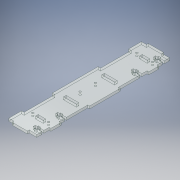
# Autodesk Inventor part: Cubierta_Rodamientos
Saved by Autodesk Inventor 2019 (Build 230136000, 136)
## iProperties
Created: 2020-04-04
Part Number: Cubierta_Rodamientos
Material: Generic
Document SubType Name: Modeling
Designer: Jurgen
Density: 1 g/cm^3
Appearance: Clear
Mass: 67.373 g
Surface Area: 309.762 cm^2
Volume: 67.373 cm^3
Author: Jurgen
Autodesk Inventor part; units mm, degrees
ref_plane "YZ Plane" through (0, 0, 0) normal (1, 0, 0) x (0, 1, 0)
ref_plane "XZ Plane" through (0, 0, 0) normal (0, 1, 0) x (-1, 0, 0)
ref_plane "XY Plane" through (0, 0, 0) normal (0, 0, 1) x (1, 0, 0)
sketch "Sketch1" plane through (0, 0, 0) normal (0, 1, 0) x (-1, 0, 0)
  line L0 (-25, -130) -> (25, -130)
  line L1 (25, 130) -> (-25, 130)
  line L2 (-25, 130) -> (-25, -130)
  line L3 (-25, -130) -> (25, 130) construction
  line L4 (25, -130) -> (-25, 130) construction
  line L5 (25, 130) -> (30, 130)
  line L6 (30, 130) -> (30, 105)
  line L7 (30, 105) -> (25, 105)
  line L8 (25, -130) -> (30, -130)
  line L9 (30, -130) -> (30, -105)
  line L10 (30, -105) -> (25, -105)
  line L11 (25, 105) -> (-25, 105) construction
  line L12 (3.2055, 0) -> (-25, 0) construction
  line L13 (25, -105) -> (-25, -105) construction
  line L14 (25, 45) -> (30, 45)
  line L15 (30, 45) -> (30, -45)
  line L16 (30, -45) -> (25, -45)
  line L17 (25, -105) -> (25, -45)
  line L18 (25, 45) -> (25, 105)
  point P0 (0, 0)
  dimension "d0" = 50
  dimension "d1" = 260
  dimension "d2" = 5
  dimension "d3" = 25
  dimension "d4" = 5
  dimension "d5" = 25
  dimension "d7" = 5
  dimension "d8" = 90
  dimension "d29" = 60
  dimension "d30" = 60
  constraints: 38 end point, 9 perpendicular, 5 parallel, 3 horizontal, 3 midpoint, 2 point on line
  measures "d0" distance of L1.end L1.start
  measures "d1" distance of L1.start L0.end
  measures "d2" distance of L7.end L6.end
  measures "d3" distance of L5.end L6.end
  measures "d4" distance of L10.end L9.end
  measures "d5" distance of L9.end L8.end
  measures "d7" distance of L14.start L14.end
  measures "d8" distance of L14.end L15.end
  measures "d29" distance of L10.end L16.end
  measures "d30" distance of L14.start L7.end
extrude "Extrusion1" add sketch "Sketch1" along normal blind 5
sketch "Sketch2" plane through (0, 5, 0) normal (0, 1, 0) x (1, 0, 0)
  line L0 (25, 130) -> (-30, 130) construction
  line L1 (-30, 130) -> (-30, 105) construction
  line L2 (-30, 105) -> (-25, 105) construction
  line L3 (-25, 105) -> (-25, 45) construction
  line L4 (-25, 45) -> (-30, 45) construction
  line L5 (-30, 45) -> (-30, -45) construction
  line L6 (-30, -45) -> (-25, -45) construction
  line L7 (-25, -45) -> (-25, -105) construction
  line L8 (-25, -105) -> (-30, -105) construction
  line L9 (-30, -105) -> (-30, -130) construction
  line L10 (-30, -130) -> (25, -130) construction
  line L11 (25, -130) -> (25, 130) construction
  line L12 (-30, 45) -> (-30, -45) construction
  line L13 (25, -130) -> (25, 130) construction
  line L14 (7.5, -100) -> (-7.5, -100)
  line L15 (-7.5, -100) -> (-7.5, -95)
  line L16 (-7.5, -95) -> (7.5, -95)
  line L17 (7.5, -95) -> (7.5, -100)
  line L18 (7.5, 109) -> (-7.5, 109)
  line L19 (-7.5, 109) -> (-7.5, 104)
  line L20 (-7.5, 104) -> (7.5, 104)
  line L21 (7.5, 104) -> (7.5, 109)
  line L22 (-7.5, 106.5) -> (25, 106.5) construction
  line L23 (-7.5, 106.5) -> (-30, 106.5) construction
  circle A0 centre (-15.5, 106.5) radius 2
  circle A1 centre (15.5, 106.5) radius 2
  line L24 (-7.5, -97.5) -> (25, -97.5) construction
  line L25 (-7.5, -97.5) -> (-25, -97.5) construction
  circle A2 centre (-15.5, -97.5) radius 2
  circle A3 centre (15.5, -97.5) radius 2
  point P0 (0, 0)
  dimension "d11" = 15
  dimension "d12" = 5
  dimension "d13" = 35
  dimension "d14" = 17.5
  dimension "d17" = 5
  dimension "d18" = 15
  dimension "d19" = 26
  dimension "d31" = 17.5
  dimension "d32" = 4
  dimension "d33" = 4
  dimension "d34" = 8
  dimension "d35" = 8
  dimension "d36" = 4
  dimension "d37" = 4
  dimension "d38" = 8
  dimension "d39" = 8
  constraints: 24 end point, 10 point on line, 4 centre point, 3 perpendicular, 2 midpoint, 2 parallel, 1 horizontal
  measures "d11" distance of L15.end L16.end
  measures "d12" distance of L14.end L15.end
  measures "d13" distance between parallel lines of L10 L16
  measures "d14" distance between parallel lines of L11 L17
  measures "d17" distance of L20.end L21.end
  measures "d18" distance of L20.start L20.end
  measures "d19" distance between parallel lines of L0 L20
  measures "d31" distance between parallel lines of L11 L21
  measures "d32" diameter of A0
  measures "d33" diameter of A1
  measures "d34" distance from line of L19 A0.centre
  measures "d35" distance from line of A1.centre L21
  measures "d36" diameter of A2
  measures "d37" diameter of A3
  measures "d38" distance from line of L15 A2.centre
  measures "d39" distance from line of A3.centre L17
extrude "Extrusion2" cut sketch "Sketch2" against normal blind 5
sketch "Sketch3" plane through (0, 5, 0) normal (0, 1, 0) x (1, 0, 0)
  line L0 (7.5, -95) -> (7.5, -100) construction
  line L1 (7.5, -100) -> (-7.5, -100) construction
  line L2 (-7.5, -100) -> (-7.5, -95) construction
  line L3 (-7.5, -95) -> (7.5, -95) construction
  line L4 (7.5, 104) -> (-7.5, 104) construction
  line L5 (-7.5, 104) -> (-7.5, 109) construction
  line L6 (-7.5, 109) -> (7.5, 109) construction
  line L7 (7.5, 109) -> (7.5, 104) construction
  line L8 (25, 130) -> (-30, 130) construction
  line L9 (-30, 130) -> (-30, 105) construction
  line L10 (-30, 105) -> (-25, 105) construction
  line L11 (-25, 105) -> (-25, 45) construction
  line L12 (-25, 45) -> (-30, 45) construction
  line L13 (-30, 45) -> (-30, -45) construction
  line L14 (-30, -45) -> (-25, -45) construction
  line L15 (-25, -45) -> (-25, -105) construction
  line L16 (-25, -105) -> (-30, -105) construction
  line L17 (-30, -105) -> (-30, -130) construction
  line L18 (-30, -130) -> (25, -130) construction
  line L19 (25, -130) -> (25, 130) construction
  circle A0 centre (-5, 15) radius 2
  circle A1 centre (-5, -15) radius 2
  line L20 (-30, 45) -> (-30, -45) construction
  line L21 (-30, 0) -> (25, 0) construction
  point P0 (0, 0)
  dimension "d20" = 4
  dimension "d21" = 4
  dimension "d23" = 15
  dimension "d24" = 15
  dimension "d25" = 25
  dimension "d26" = 25
  constraints: 2 centre point, 2 end point, 2 midpoint
  measures "d20" diameter of A0
  measures "d21" diameter of A1
  measures "d23" distance from line of A0.centre L21
  measures "d24" vertical distance of L21.start A1.centre
  measures "d25" distance from line of L13 A0.centre
  measures "d26" distance from line of A1.centre L13
extrude "Extrusion3" cut sketch "Sketch3" against normal blind 5
sketch "Sketch4" plane through (0, 5, 0) normal (0, 1, 0) x (1, 0, 0)
  circle A0 centre (-5, 15) radius 2 construction
  circle A1 centre (-5, -15) radius 2 construction
  line L0 (7.5, -95) -> (7.5, -100) construction
  line L1 (7.5, -100) -> (-7.5, -100) construction
  line L2 (-7.5, -100) -> (-7.5, -95) construction
  line L3 (-7.5, -95) -> (7.5, -95) construction
  circle A2 centre (-15.5, -97.5) radius 2 construction
  circle A3 centre (-15.5, 106.5) radius 2 construction
  circle A4 centre (15.5, 106.5) radius 2 construction
  circle A5 centre (15.5, -97.5) radius 2 construction
  line L4 (7.5, 104) -> (-7.5, 104) construction
  line L5 (-7.5, 104) -> (-7.5, 109) construction
  line L6 (-7.5, 109) -> (7.5, 109) construction
  line L7 (7.5, 109) -> (7.5, 104) construction
  line L8 (25, 130) -> (-30, 130) construction
  line L9 (-30, 130) -> (-30, 105) construction
  line L10 (-30, 105) -> (-25, 105) construction
  line L11 (-25, 105) -> (-25, 45) construction
  line L12 (-25, 45) -> (-30, 45) construction
  line L13 (-30, 45) -> (-30, -45) construction
  line L14 (-30, -45) -> (-25, -45) construction
  line L15 (-25, -45) -> (-25, -105) construction
  line L16 (-25, -105) -> (-30, -105) construction
  line L17 (-30, -105) -> (-30, -130) construction
  line L18 (-30, -130) -> (25, -130) construction
  line L19 (25, -130) -> (25, 130) construction
  line L20 (0, 0) -> (0, -130) construction
  line L21 (-30, -130) -> (25, -130) construction
  line L22 (0, 0) -> (0, 130) construction
  line L23 (25, 130) -> (-30, 130) construction
  line L24 (25, 0) -> (-30, 0) construction
  line L25 (-30, 45) -> (-30, -45) construction
  line L26 (12.5, 40) -> (-12.5, 40)
  line L27 (-12.5, 40) -> (-12.5, 35)
  line L28 (-12.5, 35) -> (12.5, 35)
  line L29 (12.5, 35) -> (12.5, 40)
  line L30 (12.5, 40) -> (-12.5, 35) construction
  line L31 (-12.5, 40) -> (12.5, 35) construction
  line L32 (12.5, -40) -> (-12.5, -40)
  line L33 (-12.5, -40) -> (-12.5, -35)
  line L34 (-12.5, -35) -> (12.5, -35)
  line L35 (12.5, -35) -> (12.5, -40)
  line L36 (12.5, -40) -> (-12.5, -35) construction
  line L37 (-12.5, -40) -> (12.5, -35) construction
  point P0 (0, 37.5)
  point P1 (0, -37.5)
  dimension "d42" = 25
  dimension "d43" = 5
  dimension "d44" = 90
  constraints: 30 end point, 6 midpoint, 5 symmetric about line, 4 point on line, 2 parallel, 2 perpendicular, 1 horizontal
  measures "d42" distance of L28.end L27.end
  measures "d43" distance of L27.end L26.end
  measures "d44" distance between parallel lines of L8 L26
extrude "Extrusion4" cut sketch "Sketch4" against normal blind 10
sketch "Sketch5" plane through (0, 5, 0) normal (0, 1, 0) x (1, 0, 0)
  line L0 (-12.5, 35) -> (-12.5, 40) construction
  line L1 (-12.5, 40) -> (12.5, 40) construction
  line L2 (12.5, 40) -> (12.5, 35) construction
  line L3 (12.5, 35) -> (-12.5, 35) construction
  line L4 (12.5, -40) -> (-12.5, -40) construction
  line L5 (-12.5, -40) -> (-12.5, -35) construction
  line L6 (-12.5, -35) -> (12.5, -35) construction
  line L7 (12.5, -35) -> (12.5, -40) construction
  circle A0 centre (-5, 15) radius 2 construction
  circle A1 centre (-5, -15) radius 2 construction
  line L8 (7.5, -95) -> (7.5, -100) construction
  line L9 (7.5, -100) -> (-7.5, -100) construction
  line L10 (-7.5, -100) -> (-7.5, -95) construction
  line L11 (-7.5, -95) -> (7.5, -95) construction
  circle A2 centre (-15.5, -97.5) radius 2 construction
  circle A3 centre (-15.5, 106.5) radius 2 construction
  circle A4 centre (15.5, 106.5) radius 2 construction
  circle A5 centre (15.5, -97.5) radius 2 construction
  line L12 (7.5, 104) -> (-7.5, 104) construction
  line L13 (-7.5, 104) -> (-7.5, 109) construction
  line L14 (-7.5, 109) -> (7.5, 109) construction
  line L15 (7.5, 109) -> (7.5, 104) construction
  line L16 (25, 130) -> (-30, 130) construction
  line L17 (-30, 130) -> (-30, 105) construction
  line L18 (-30, 105) -> (-25, 105) construction
  line L19 (-25, 105) -> (-25, 45) construction
  line L20 (-25, 45) -> (-30, 45) construction
  line L21 (-30, 45) -> (-30, -45) construction
  line L22 (-30, -45) -> (-25, -45) construction
  line L23 (-25, -45) -> (-25, -105) construction
  line L24 (-25, -105) -> (-30, -105) construction
  line L25 (-30, -105) -> (-30, -130) construction
  line L26 (-30, -130) -> (25, -130) construction
  line L27 (25, -130) -> (25, 130) construction
  line L28 (0, -40) -> (0, -45) construction
  line L29 (0, -45) -> (-20, -45) construction
  line L30 (-20, -45) -> (-20, -40) construction
  line L31 (-20, -40) -> (0, -40) construction
  line L32 (0, 45) -> (0, 40) construction
  line L33 (0, 40) -> (-20, 40) construction
  line L34 (-20, 40) -> (-20, 45) construction
  line L35 (-20, 45) -> (0, 45) construction
  circle A6 centre (-30.5, 97.5) radius 2 construction
  circle A7 centre (-30.5, -106.5) radius 2 construction
  circle A8 centre (10.5, -106.5) radius 2 construction
  circle A9 centre (10.5, 97.5) radius 2 construction
  line L36 (-22.5, 95) -> (-22.5, 100) construction
  line L37 (-22.5, 100) -> (2.5, 100) construction
  line L38 (2.5, 100) -> (2.5, 95) construction
  line L39 (2.5, 95) -> (-22.5, 95) construction
  line L40 (2.5, -109) -> (-22.5, -109) construction
  line L41 (-22.5, -109) -> (-22.5, -104) construction
  line L42 (-22.5, -104) -> (2.5, -104) construction
  line L43 (2.5, -104) -> (2.5, -109) construction
  line L44 (-50, -130) -> (25, -130) construction
  line L45 (25, -130) -> (25, 130) construction
  line L46 (25, 130) -> (-50, 130) construction
  line L47 (-50, 130) -> (-50, 105) construction
  line L48 (-50, 105) -> (-45, 105) construction
  line L49 (-45, 105) -> (-45, 45) construction
  line L50 (-45, 45) -> (-50, 45) construction
  line L51 (-50, 45) -> (-50, -45) construction
  line L52 (-50, -45) -> (-45, -45) construction
  line L53 (-45, -45) -> (-45, -105) construction
  line L54 (-45, -105) -> (-50, -105) construction
  line L55 (-50, -105) -> (-50, -130) construction
  line L56 (25, -130) -> (25, 130) construction
  line L57 (25, -120) -> (10, -120) construction
  line L58 (10, -120) -> (10, -116) construction
  line L59 (10, -116) -> (25, -116) construction
  line L60 (25, -116) -> (25, -120) construction
  line L61 (10, -118) -> (25, -118) construction
  line L62 (18, -114) -> (14, -114) construction
  line L63 (14, -114) -> (14, -122) construction
  line L64 (14, -122) -> (18, -122) construction
  line L65 (18, -122) -> (18, -114) construction
  line L66 (18, -114) -> (14, -122) construction
  line L67 (14, -114) -> (18, -122) construction
  line L68 (25, -116) -> (25, -120)
  line L69 (25, -120) -> (18, -120)
  line L70 (18, -120) -> (18, -122)
  line L71 (18, -122) -> (14, -122)
  line L72 (14, -122) -> (14, -120)
  line L73 (14, -120) -> (10, -120)
  line L74 (10, -120) -> (10, -116)
  line L75 (10, -116) -> (14, -116)
  line L76 (14, -116) -> (14, -114)
  line L77 (14, -114) -> (18, -114)
  line L78 (18, -114) -> (18, -116)
  line L79 (18, -116) -> (25, -116)
  line L80 (18, -70) -> (14, -70) construction
  line L81 (14, -70) -> (18, -70)
  line L82 (18, -70) -> (18, -72)
  line L83 (10, -72) -> (25, -72) construction
  line L84 (10, -74) -> (25, -74) construction
  line L85 (25, -76) -> (10, -76) construction
  line L86 (18, -78) -> (18, -70) construction
  line L87 (18, -70) -> (14, -78) construction
  line L88 (14, -70) -> (18, -78) construction
  line L89 (14, -70) -> (14, -78) construction
  line L90 (14, -78) -> (18, -78) construction
  line L91 (18, -78) -> (14, -78)
  line L92 (18, -76) -> (18, -78)
  line L93 (25, -76) -> (18, -76)
  line L94 (25, -72) -> (25, -76) construction
  line L95 (25, -72) -> (25, -76)
  line L96 (18, -72) -> (25, -72)
  line L97 (10, -76) -> (10, -72) construction
  line L98 (14, -78) -> (14, -76)
  line L99 (14, -72) -> (14, -70)
  line L100 (10, -72) -> (14, -72)
  line L101 (14, -76) -> (10, -76)
  line L102 (10, -76) -> (10, -72)
  line L103 (25, -106) -> (28.5, -106)
  line L104 (28.5, -106) -> (28.5, -86)
  line L105 (28.5, -86) -> (25, -86)
  line L106 (25, -86) -> (25, -106)
  line L107 (25, 106) -> (25, 86)
  line L108 (28.5, 106) -> (25, 106)
  line L109 (28.5, 86) -> (28.5, 106)
  line L110 (25, 86) -> (28.5, 86)
  line L111 (10, 72) -> (10, 76) construction
  line L112 (10, 72) -> (10, 76)
  line L113 (14, 76) -> (14, 78)
  line L114 (10, 76) -> (14, 76)
  line L115 (14, 72) -> (10, 72)
  line L116 (14, 70) -> (14, 72)
  line L117 (14, 78) -> (14, 70) construction
  line L118 (18, 72) -> (18, 70)
  line L119 (18, 70) -> (18, 78) construction
  line L120 (18, 70) -> (14, 70)
  line L121 (18, 78) -> (14, 70) construction
  line L122 (14, 78) -> (18, 70) construction
  line L123 (14, 70) -> (18, 70) construction
  line L124 (18, 78) -> (18, 76)
  line L125 (18, 78) -> (14, 78) construction
  line L126 (10, 76) -> (25, 76) construction
  line L127 (10, 74) -> (25, 74) construction
  line L128 (25, 72) -> (10, 72) construction
  line L129 (14, 78) -> (18, 78)
  line L130 (18, 122) -> (14, 122) construction
  line L131 (14, 122) -> (18, 122)
  line L132 (18, 122) -> (18, 120)
  line L133 (10, 118) -> (25, 118) construction
  line L134 (25, 116) -> (10, 116) construction
  line L135 (10, 120) -> (25, 120) construction
  line L136 (14, 114) -> (18, 114) construction
  line L137 (18, 114) -> (14, 114)
  line L138 (14, 114) -> (14, 116)
  line L139 (14, 116) -> (10, 116)
  line L140 (10, 120) -> (14, 120)
  line L141 (10, 116) -> (10, 120)
  line L142 (10, 116) -> (10, 120) construction
  line L143 (18, 114) -> (18, 122) construction
  line L144 (18, 122) -> (14, 114) construction
  line L145 (14, 122) -> (14, 114) construction
  line L146 (14, 120) -> (14, 122)
  line L147 (14, 122) -> (18, 114) construction
  line L148 (18, 76) -> (25, 76)
  line L149 (25, 76) -> (25, 72) construction
  line L150 (25, 76) -> (25, 72)
  line L151 (25, 72) -> (18, 72)
  line L152 (25, 120) -> (25, 116) construction
  line L153 (25, 120) -> (25, 116)
  line L154 (18, 120) -> (25, 120)
  line L155 (25, 116) -> (18, 116)
  line L156 (18, 116) -> (18, 114)
  line L157 (25, -30) -> (28.5, -30)
  line L158 (28.5, -30) -> (28.5, 30)
  line L159 (28.5, 30) -> (25, 30)
  line L160 (25, 30) -> (25, -30)
  line L161 (25, -130) -> (25, 130)
  point P0 (0, 0)
  point P1 (0, 0)
  point P2 (16, -118)
  point P3 (16, -74)
  point P4 (16, 74)
  point P5 (16, 118)
  dimension "d47" = 15
  dimension "d48" = 4
  dimension "d49" = 4
  dimension "d50" = 8
  dimension "d51" = 4
  dimension "d52" = 10
  dimension "d53" = 15
  dimension "d54" = 4
  dimension "d55" = 4
  dimension "d56" = 8
  dimension "d57" = 4
  dimension "d58" = 40
  dimension "d59" = 3.5
  dimension "d60" = 20
  dimension "d61" = 10
  dimension "d62" = 15
  dimension "d63" = 4
  dimension "d64" = 4
  dimension "d65" = 8
  dimension "d66" = 4
  dimension "d67" = 15
  dimension "d68" = 4
  dimension "d69" = 4
  dimension "d70" = 8
  dimension "d71" = 4
  dimension "d72" = 40
  dimension "d73" = 3.5
  dimension "d74" = 20
  dimension "d75" = 10
  dimension "d76" = 10
  dimension "d77" = 3.5
  dimension "d78" = 60
  dimension "d79" = 30
  constraints: 266 end point, 39 point on line, 23 perpendicular, 22 parallel, 16 midpoint, 11 horizontal, 9 collinear, 4 centre point, 1 vertical, 3 other
  measures "d47" distance of L58.end L59.end
  measures "d48" distance of L57.end L58.end
  measures "d49" distance of L64.end L63.end
  measures "d50" distance of L63.end L62.end
  measures "d51" distance between parallel lines of L58 L63
  measures "d52" distance between parallel lines of L44 L57
  measures "d53" distance of L83.start L83.end
  measures "d54" distance of L85.end L83.start
  measures "d55" distance of L86.start L87.end
  measures "d56" distance of L87.end L80.end
  measures "d57" distance between parallel lines of L97 L89
  measures "d58" distance between parallel lines of L79 L93
  measures "d59" distance of L105.end L104.end
  measures "d60" distance of L104.end L103.end
  measures "d61" distance between parallel lines of L59 L103
  measures "d62" distance of L111.end L126.end
  measures "d63" distance of L111.start L111.end
  measures "d64" distance of L118.end L116.start
  measures "d65" distance of L116.start L113.end
  measures "d66" distance between parallel lines of L111 L117
  measures "d67" distance of L135.start L135.end
  measures "d68" distance of L134.end L135.start
  measures "d69" distance of L136.end L136.start
  measures "d70" distance of L136.start L130.end
  measures "d71" distance between parallel lines of L142 L145
  measures "d72" distance between parallel lines of L148 L155
  measures "d73" distance of L107.start L108.start
  measures "d74" distance of L108.start L109.start
  measures "d75" distance between parallel lines of L126 L110
  measures "d76" distance between parallel lines of L46 L154
  measures "d77" distance of L159.end L158.end
  measures "d78" distance of L158.end L157.end
  measures "d79" distance from line of point (0, 0) L157
extrude "Extrusion5" add sketch "Sketch5" against normal blind 5 contours L107 L108 L109 L110 | L160 L159 L158 L157 | L106 L105 L104 L103
sketch "Sketch6" plane through (0, 5, 0) normal (0, 1, 0) x (1, 0, 0)
  line L0 (-12.5, 35) -> (-12.5, 40) construction
  line L1 (-12.5, 40) -> (12.5, 40) construction
  line L2 (12.5, 40) -> (12.5, 35) construction
  line L3 (12.5, 35) -> (-12.5, 35) construction
  line L4 (12.5, -40) -> (-12.5, -40) construction
  line L5 (-12.5, -40) -> (-12.5, -35) construction
  line L6 (-12.5, -35) -> (12.5, -35) construction
  line L7 (12.5, -35) -> (12.5, -40) construction
  circle A0 centre (-5, 15) radius 2 construction
  circle A1 centre (-5, -15) radius 2 construction
  line L8 (7.5, -95) -> (7.5, -100) construction
  line L9 (7.5, -100) -> (-7.5, -100) construction
  line L10 (-7.5, -100) -> (-7.5, -95) construction
  line L11 (-7.5, -95) -> (7.5, -95) construction
  circle A2 centre (-15.5, -97.5) radius 2 construction
  circle A3 centre (-15.5, 106.5) radius 2 construction
  circle A4 centre (15.5, 106.5) radius 2 construction
  circle A5 centre (15.5, -97.5) radius 2 construction
  line L12 (7.5, 104) -> (-7.5, 104) construction
  line L13 (-7.5, 104) -> (-7.5, 109) construction
  line L14 (-7.5, 109) -> (7.5, 109) construction
  line L15 (7.5, 109) -> (7.5, 104) construction
  line L16 (25, 130) -> (-30, 130) construction
  line L17 (-30, 130) -> (-30, 105) construction
  line L18 (-30, 105) -> (-25, 105) construction
  line L19 (-25, 105) -> (-25, 45) construction
  line L20 (-25, 45) -> (-30, 45) construction
  line L21 (-30, 45) -> (-30, -45) construction
  line L22 (-30, -45) -> (-25, -45) construction
  line L23 (-25, -45) -> (-25, -105) construction
  line L24 (-25, -105) -> (-30, -105) construction
  line L25 (-30, -105) -> (-30, -130) construction
  line L26 (-30, -130) -> (25, -130) construction
  line L27 (25, -130) -> (25, -106) construction
  line L28 (25, -106) -> (28.5, -106) construction
  line L29 (28.5, -106) -> (28.5, -86) construction
  line L30 (28.5, -86) -> (25, -86) construction
  line L31 (25, -86) -> (25, -30) construction
  line L32 (25, -30) -> (28.5, -30) construction
  line L33 (28.5, -30) -> (28.5, 30) construction
  line L34 (28.5, 30) -> (25, 30) construction
  line L35 (25, 30) -> (25, 86) construction
  line L36 (28.5, 86) -> (25, 86) construction
  line L37 (28.5, 106) -> (28.5, 86) construction
  line L38 (25, 106) -> (28.5, 106) construction
  line L39 (25, 106) -> (25, 130) construction
  line L40 (0, -40) -> (0, -45) construction
  line L41 (0, -45) -> (-20, -45) construction
  line L42 (-20, -45) -> (-20, -40) construction
  line L43 (-20, -40) -> (0, -40) construction
  line L44 (0, 45) -> (0, 40) construction
  line L45 (0, 40) -> (-20, 40) construction
  line L46 (-20, 40) -> (-20, 45) construction
  line L47 (-20, 45) -> (0, 45) construction
  circle A6 centre (-30.5, 97.5) radius 2 construction
  circle A7 centre (-30.5, -106.5) radius 2 construction
  circle A8 centre (10.5, -106.5) radius 2 construction
  circle A9 centre (10.5, 97.5) radius 2 construction
  line L48 (-22.5, 95) -> (-22.5, 100) construction
  line L49 (-22.5, 100) -> (2.5, 100) construction
  line L50 (2.5, 100) -> (2.5, 95) construction
  line L51 (2.5, 95) -> (-22.5, 95) construction
  line L52 (2.5, -109) -> (-22.5, -109) construction
  line L53 (-22.5, -109) -> (-22.5, -104) construction
  line L54 (-22.5, -104) -> (2.5, -104) construction
  line L55 (2.5, -104) -> (2.5, -109) construction
  line L56 (-50, -130) -> (25, -130) construction
  line L57 (25, -130) -> (25, -106) construction
  line L58 (25, -106) -> (30.5, -106) construction
  line L59 (30.5, -106) -> (30.5, -86) construction
  line L60 (30.5, -86) -> (23, -86) construction
  line L61 (23, -86) -> (23, -30) construction
  line L62 (23, -30) -> (26.5, -30) construction
  line L63 (26.5, -30) -> (26.5, 30) construction
  line L64 (26.5, 30) -> (23, 30) construction
  line L65 (23, 30) -> (23, 86) construction
  line L66 (26.5, 86) -> (23, 86) construction
  line L67 (26.5, 106) -> (26.5, 86) construction
  line L68 (23, 106) -> (26.5, 106) construction
  line L69 (23, 106) -> (23, 130) construction
  line L70 (23, 130) -> (-50, 130) construction
  line L71 (-50, 130) -> (-50, 105) construction
  line L72 (-50, 105) -> (-45, 105) construction
  line L73 (-45, 105) -> (-45, 45) construction
  line L74 (-45, 45) -> (-50, 45) construction
  line L75 (-50, 45) -> (-50, -45) construction
  line L76 (-50, -45) -> (-45, -45) construction
  line L77 (-45, -45) -> (-45, -105) construction
  line L78 (-45, -105) -> (-50, -105) construction
  line L79 (-50, -105) -> (-50, -130) construction
  line L80 (25, -130) -> (25, -106) construction
  line L81 (25, -120) -> (8, -120) construction
  line L82 (8, -120) -> (8, -116) construction
  line L83 (8, -116) -> (25, -116) construction
  line L84 (25, -116) -> (25, -120) construction
  line L85 (8, -118) -> (25, -118) construction
  line L86 (16, -122) -> (12, -122) construction
  line L87 (12, -122) -> (12, -114) construction
  line L88 (12, -114) -> (16, -114) construction
  line L89 (16, -114) -> (16, -122) construction
  line L90 (16, -122) -> (12, -114) construction
  line L91 (12, -122) -> (16, -114) construction
  line L92 (25, -120) -> (16, -120)
  line L93 (16, -120) -> (16, -122)
  line L94 (16, -122) -> (12, -122)
  line L95 (12, -122) -> (12, -120)
  line L96 (12, -120) -> (8, -120)
  line L97 (8, -120) -> (8, -116)
  line L98 (8, -116) -> (12, -116)
  line L99 (12, -116) -> (12, -114)
  line L100 (12, -114) -> (16, -114)
  line L101 (16, -114) -> (16, -116)
  line L102 (16, -116) -> (25, -116)
  line L103 (25, -120) -> (25, -116)
  line L104 (16, -76) -> (16, -78)
  line L105 (16, -78) -> (12, -78)
  line L106 (12, -78) -> (12, -76)
  line L107 (16, -78) -> (12, -78) construction
  line L108 (16, -70) -> (16, -72)
  line L109 (25, -76) -> (16, -76)
  line L110 (12, -70) -> (16, -70) construction
  line L111 (12, -70) -> (16, -70)
  line L112 (12, -72) -> (12, -70)
  line L113 (16, -70) -> (16, -78) construction
  line L114 (12, -76) -> (8, -76)
  line L115 (12, -78) -> (16, -70) construction
  line L116 (12, -78) -> (12, -70) construction
  line L117 (16, -78) -> (12, -70) construction
  line L118 (8, -72) -> (12, -72)
  line L119 (8, -76) -> (8, -72)
  line L120 (25, -76) -> (8, -76) construction
  line L121 (8, -72) -> (25, -72) construction
  line L122 (8, -74) -> (25, -74) construction
  line L123 (16, -72) -> (25, -72)
  line L124 (25, -76) -> (25, -72)
  line L125 (25, -72) -> (25, -76) construction
  line L126 (8, -76) -> (8, -72) construction
  line L127 (16, 72) -> (16, 70)
  line L128 (16, 70) -> (12, 70)
  line L129 (12, 70) -> (12, 72)
  line L130 (16, 70) -> (12, 70) construction
  line L131 (16, 78) -> (16, 76)
  line L132 (25, 72) -> (16, 72)
  line L133 (12, 78) -> (16, 78) construction
  line L134 (12, 78) -> (16, 78)
  line L135 (12, 76) -> (12, 78)
  line L136 (16, 78) -> (16, 70) construction
  line L137 (12, 72) -> (8, 72)
  line L138 (12, 70) -> (16, 78) construction
  line L139 (12, 70) -> (12, 78) construction
  line L140 (16, 70) -> (12, 78) construction
  line L141 (8, 76) -> (12, 76)
  line L142 (8, 72) -> (8, 76)
  line L143 (25, 72) -> (8, 72) construction
  line L144 (8, 76) -> (25, 76) construction
  line L145 (8, 74) -> (25, 74) construction
  line L146 (16, 76) -> (25, 76)
  line L147 (25, 72) -> (25, 76)
  line L148 (25, 76) -> (25, 72) construction
  line L149 (8, 72) -> (8, 76) construction
  line L150 (16, 116) -> (16, 114)
  line L151 (16, 114) -> (12, 114)
  line L152 (12, 114) -> (12, 116)
  line L153 (16, 114) -> (12, 114) construction
  line L154 (16, 122) -> (16, 120)
  line L155 (25, 116) -> (16, 116)
  line L156 (12, 122) -> (16, 122) construction
  line L157 (12, 122) -> (16, 122)
  line L158 (12, 120) -> (12, 122)
  line L159 (16, 122) -> (16, 114) construction
  line L160 (12, 116) -> (8, 116)
  line L161 (12, 114) -> (16, 122) construction
  line L162 (12, 114) -> (12, 122) construction
  line L163 (16, 114) -> (12, 122) construction
  line L164 (8, 120) -> (12, 120)
  line L165 (8, 116) -> (8, 120)
  line L166 (25, 116) -> (8, 116) construction
  line L167 (8, 120) -> (25, 120) construction
  line L168 (8, 118) -> (25, 118) construction
  line L169 (16, 120) -> (25, 120)
  line L170 (25, 116) -> (25, 120)
  line L171 (25, 120) -> (25, 116) construction
  line L172 (8, 116) -> (8, 120) construction
  point P0 (0, 0)
  point P1 (14, -118)
  point P2 (14, -74)
  point P3 (14, 74)
  point P4 (14, 118)
  dimension "d82" = 17
  dimension "d83" = 4
  dimension "d84" = 4
  dimension "d85" = 8
  dimension "d86" = 10
  dimension "d87" = 17
  dimension "d88" = 4
  dimension "d89" = 4
  dimension "d90" = 8
  dimension "d91" = 17
  dimension "d92" = 4
  dimension "d93" = 4
  dimension "d94" = 8
  dimension "d95" = 17
  dimension "d96" = 4
  dimension "d97" = 4
  dimension "d98" = 8
  dimension "d99" = 10
  dimension "d100" = 10
  dimension "d101" = 10
  dimension "d112" = 0
  dimension "d113" = 0
  dimension "d114" = 4
  dimension "d115" = 4
  dimension "d116" = 0
  dimension "d117" = 4
  dimension "d118" = 0
  dimension "d119" = 4
  constraints: 266 end point, 41 point on line, 28 perpendicular, 16 midpoint, 16 parallel, 8 collinear, 8 horizontal, 4 centre point
  measures "d82" distance of L82.end L83.end
  measures "d83" distance of L81.end L82.end
  measures "d84" distance of L87.end L88.end
  measures "d85" distance of L86.end L87.end
  measures "d86" distance between parallel lines of L56 L81
  measures "d87" distance of L118.start L121.end
  measures "d88" distance of L114.end L118.start
  measures "d89" distance of L110.start L108.start
  measures "d90" distance of L105.end L110.start
  measures "d91" distance of L141.start L144.end
  measures "d92" distance of L137.end L141.start
  measures "d93" distance of L133.start L131.start
  measures "d94" distance of L128.end L133.start
  measures "d95" distance of L164.start L167.end
  measures "d96" distance of L160.end L164.start
  measures "d97" distance of L156.start L154.start
  measures "d98" distance of L151.end L156.start
  measures "d99" distance between parallel lines of L120 L60
  measures "d100" distance between parallel lines of L66 L144
  measures "d101" distance between parallel lines of L68 L166
  measures "d112" distance between parallel lines of L27 L57
  measures "d113" distance between parallel lines of L31 L124
  measures "d114" distance between parallel lines of L119 L112
  measures "d115" distance between parallel lines of L82 L87
  measures "d116" distance between parallel lines of L35 L147
  measures "d117" distance between parallel lines of L149 L135
  measures "d118" distance between parallel lines of L39 L170
  measures "d119" distance between parallel lines of L162 L165
extrude "Extrusion6" cut sketch "Sketch6" against normal blind 5
sketch "Sketch7" plane through (0, 5, 0) normal (0, 1, 0) x (1, 0, 0)
  line L0 (16, 76) -> (25, 76) construction
  line L1 (25, 76) -> (25, 86) construction
  line L2 (28.5, 86) -> (25, 86) construction
  line L3 (28.5, 106) -> (28.5, 86) construction
  line L4 (25, 106) -> (28.5, 106) construction
  line L5 (25, 106) -> (25, 116) construction
  line L6 (25, 116) -> (16, 116) construction
  line L7 (16, 116) -> (16, 114) construction
  line L8 (16, 114) -> (12, 114) construction
  line L9 (12, 114) -> (12, 116) construction
  line L10 (12, 116) -> (8, 116) construction
  line L11 (8, 116) -> (8, 120) construction
  line L12 (8, 120) -> (12, 120) construction
  line L13 (12, 120) -> (12, 122) construction
  line L14 (12, 122) -> (16, 122) construction
  line L15 (16, 122) -> (16, 120) construction
  line L16 (16, 120) -> (25, 120) construction
  line L17 (25, 120) -> (25, 130) construction
  line L18 (25, 130) -> (-30, 130) construction
  line L19 (-30, 130) -> (-30, 105) construction
  line L20 (-30, 105) -> (-25, 105) construction
  line L21 (-25, 105) -> (-25, 45) construction
  line L22 (-25, 45) -> (-30, 45) construction
  line L23 (-30, 45) -> (-30, -45) construction
  line L24 (-30, -45) -> (-25, -45) construction
  line L25 (-25, -45) -> (-25, -105) construction
  line L26 (-25, -105) -> (-30, -105) construction
  line L27 (-30, -105) -> (-30, -130) construction
  line L28 (-30, -130) -> (25, -130) construction
  line L29 (25, -130) -> (25, -120) construction
  line L30 (25, -120) -> (16, -120) construction
  line L31 (16, -120) -> (16, -122) construction
  line L32 (16, -122) -> (12, -122) construction
  line L33 (12, -122) -> (12, -120) construction
  line L34 (12, -120) -> (8, -120) construction
  line L35 (8, -120) -> (8, -116) construction
  line L36 (8, -116) -> (12, -116) construction
  line L37 (12, -116) -> (12, -114) construction
  line L38 (12, -114) -> (16, -114) construction
  line L39 (16, -114) -> (16, -116) construction
  line L40 (16, -116) -> (25, -116) construction
  line L41 (25, -116) -> (25, -106) construction
  line L42 (25, -106) -> (28.5, -106) construction
  line L43 (28.5, -106) -> (28.5, -86) construction
  line L44 (28.5, -86) -> (25, -86) construction
  line L45 (25, -86) -> (25, -76) construction
  line L46 (25, -76) -> (16, -76) construction
  line L47 (16, -76) -> (16, -78) construction
  line L48 (16, -78) -> (12, -78) construction
  line L49 (12, -78) -> (12, -76) construction
  line L50 (12, -76) -> (8, -76) construction
  line L51 (8, -76) -> (8, -72) construction
  line L52 (8, -72) -> (12, -72) construction
  line L53 (12, -72) -> (12, -70) construction
  line L54 (12, -70) -> (16, -70) construction
  line L55 (16, -70) -> (16, -72) construction
  line L56 (16, -72) -> (25, -72) construction
  line L57 (25, -72) -> (25, -30) construction
  line L58 (25, -30) -> (28.5, -30) construction
  line L59 (28.5, -30) -> (28.5, 30) construction
  line L60 (28.5, 30) -> (25, 30) construction
  line L61 (25, 30) -> (25, 72) construction
  line L62 (25, 72) -> (16, 72) construction
  line L63 (16, 72) -> (16, 70) construction
  line L64 (16, 70) -> (12, 70) construction
  line L65 (12, 70) -> (12, 72) construction
  line L66 (12, 72) -> (8, 72) construction
  line L67 (8, 72) -> (8, 76) construction
  line L68 (8, 76) -> (12, 76) construction
  line L69 (12, 76) -> (12, 78) construction
  line L70 (12, 78) -> (16, 78) construction
  line L71 (16, 78) -> (16, 76) construction
  line L72 (-12.5, 35) -> (-12.5, 40) construction
  line L73 (-12.5, 40) -> (12.5, 40) construction
  line L74 (12.5, 40) -> (12.5, 35) construction
  line L75 (12.5, 35) -> (-12.5, 35) construction
  line L76 (12.5, -40) -> (-12.5, -40) construction
  line L77 (-12.5, -40) -> (-12.5, -35) construction
  line L78 (-12.5, -35) -> (12.5, -35) construction
  line L79 (12.5, -35) -> (12.5, -40) construction
  circle A0 centre (-5, 15) radius 2 construction
  circle A1 centre (-5, -15) radius 2 construction
  line L80 (7.5, -95) -> (7.5, -100) construction
  line L81 (7.5, -100) -> (-7.5, -100) construction
  line L82 (-7.5, -100) -> (-7.5, -95) construction
  line L83 (-7.5, -95) -> (7.5, -95) construction
  circle A2 centre (-15.5, -97.5) radius 2 construction
  circle A3 centre (-15.5, 106.5) radius 2 construction
  circle A4 centre (15.5, 106.5) radius 2 construction
  circle A5 centre (15.5, -97.5) radius 2 construction
  line L84 (7.5, 104) -> (-7.5, 104) construction
  line L85 (-7.5, 104) -> (-7.5, 109) construction
  line L86 (-7.5, 109) -> (7.5, 109) construction
  line L87 (7.5, 109) -> (7.5, 104) construction
  line L88 (-20, -130) -> (10, -130)
  line L89 (10, -130) -> (10, -133.5)
  line L90 (10, -133.5) -> (-20, -133.5)
  line L91 (-20, -133.5) -> (-20, -130)
  line L92 (25, 130) -> (-30, 130) construction
  line L93 (-20, 130) -> (10, 130)
  line L94 (10, 130) -> (10, 133.5)
  line L95 (10, 133.5) -> (-20, 133.5)
  line L96 (-20, 133.5) -> (-20, 130)
  point P0 (0, 0)
  dimension "d104" = 30
  dimension "d105" = 3.5
  dimension "d106" = 10
  dimension "d107" = 30
  dimension "d108" = 3.5
  dimension "d109" = 10
  constraints: 16 end point, 4 parallel, 2 horizontal, 2 perpendicular, 2 point on line
  measures "d104" distance of L89.end L90.end
  measures "d105" distance of L88.end L89.end
  measures "d106" distance between parallel lines of L27 L91
  measures "d107" distance of L95.end L94.end
  measures "d108" distance of L94.end L93.end
  measures "d109" distance between parallel lines of L96 L19
extrude "Extrusion7" add sketch "Sketch7" against normal blind 5
body "Solid1"
